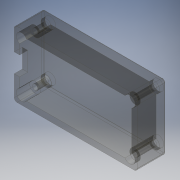
# Autodesk Inventor part: sevo onder
Saved by Autodesk Inventor 2019 (Build 230136000, 136)
## iProperties
Created: 2021-01-16
Part Number: sevo onder
Material: Glass
Document SubType Name: Modeling
Designer: CS
Density: 2.18 g/cm^3
Appearance: Clear servo black(1)
Author: CS
Autodesk Inventor part; units mm, degrees
ref_plane "YZ Plane" through (0, 0, 0) normal (1, 0, 0) x (0, 1, 0)
ref_plane "XZ Plane" through (0, 0, 0) normal (0, 1, 0) x (-1, 0, 0)
ref_plane "XY Plane" through (0, 0, 0) normal (0, 0, 1) x (1, 0, 0)
sketch "Sketch1" plane through (0, 0, 0) normal (0, 0, 1) x (1, 0, 0)
  line L0 (11.375, -6.1) -> (-11.375, -6.1)
  line L1 (-11.375, -6.1) -> (-11.375, 6.1)
  line L2 (-11.375, 6.1) -> (11.375, 6.1)
  line L3 (11.375, 6.1) -> (11.375, -6.1)
  line L4 (11.375, -6.1) -> (-11.375, 6.1) construction
  line L5 (-11.375, -6.1) -> (11.375, 6.1) construction
  point P0 (0, 0)
  dimension "d0" = 12.2
  dimension "d1" = 22.75
  constraints: 12 end point, 2 midpoint, 2 parallel, 1 horizontal, 1 perpendicular
  measures "d0" distance of L2.end L0.start
  measures "d1" distance of L1.end L2.end
extrude "Extrusion1" add sketch "Sketch1" along normal blind 5.3
fillet "Fillet1" radius 0.5 4 edges at (-11.375, 6.1, 2.65) (-11.375, -6.1, 2.65) (11.375, -6.1, 2.65) (11.375, 6.1, 2.65)
fillet "Fillet1" radius 0.25 4 edges at (0, -6.1, 0) (-11.375, 0, 0) (0, 6.1, 0) (11.375, 0, 0)
sketch "Sketch2" plane through (0, 0, 5.3) normal (0, 0, 1) x (1, 0, 0)
  line L0 (10.375, -5) -> (-10.375, -5)
  line L1 (-10.375, -5) -> (-10.375, 5)
  line L2 (-10.375, 5) -> (10.375, 5)
  line L3 (10.375, 5) -> (10.375, -5)
  line L4 (10.375, -5) -> (-10.375, 5) construction
  line L5 (-10.375, -5) -> (10.375, 5) construction
  line L6 (10.875, 6.1) -> (-10.875, 6.1) projected
  line L7 (-11.375, 5.6) -> (-11.375, -5.6) projected
  line L8 (-11.375, -5.6) -> (-11.375, 5.6) projected
  line L9 (-10.375, -1.75) -> (-11.375, -1.75)
  line L10 (-11.375, -1.75) -> (-11.375, 1.75)
  line L11 (-11.375, 1.75) -> (-10.375, 1.75)
  line L12 (-10.375, 1.75) -> (-10.375, -1.75)
  line L13 (10, -4.5) -> (-10, -4.5) construction
  line L14 (-10, -4.5) -> (-10, 4.5) construction
  line L15 (-10, 4.5) -> (10, 4.5) construction
  line L16 (10, 4.5) -> (10, -4.5) construction
  line L17 (10, -4.5) -> (-10, 4.5) construction
  line L18 (-10, -4.5) -> (10, 4.5) construction
  circle A0 centre (-10, 4.5) radius 0.5
  circle A1 centre (10, 4.5) radius 0.5
  circle A2 centre (-10, -4.5) radius 0.5
  circle A3 centre (10, -4.5) radius 0.5
  circle A4 centre (-10, 4.5) radius 1
  circle A5 centre (10, 4.5) radius 1
  circle A6 centre (-10, -4.5) radius 1
  circle A7 centre (10, -4.5) radius 1
  point P0 (0, 0)
  point P1 (-11.375, 0)
  point P2 (0, 0)
  point P3 (-11.375, 0)
  point P4 (0, 0)
  dimension "d6" = 1.1
  dimension "d7" = 1
  dimension "d8" = 3.5
  dimension "d9" = 20
  dimension "d10" = 9
  dimension "d11" = 1
  dimension "d12" = 2
  constraints: 32 end point, 8 centre point, 8 coincident, 8 midpoint, 6 equal radius, 6 parallel, 3 horizontal, 3 perpendicular, 2 horizontal alignment, 2 point on line
  measures "d6" distance between parallel lines of L6 L2
  measures "d7" distance between parallel lines of L7 L1
  measures "d8" distance between parallel lines of L9 L11
  measures "d9" distance of L14.end L15.end
  measures "d10" distance of L15.end L13.start
  measures "d11" diameter of A0
  measures "d12" diameter of A4
extrude "Extrusion2" cut sketch "Sketch2" against normal blind 4.5 contours L0 A3 L3 | L0 A7 L3 A3 | A3 L3 | L0 A6 L1 A4 L2 A5 L3 A7 | L0 A2 L1 A6 | L0 L1 A2 | A2 L1 | A5 L2 A1 L3 | A1 L3 | A1 L2 L3 | A4 L1 A0 L2 | A0 L1 L2 | A0 L1 picked at (10.2274, -3.7042) picked at (10.11, -4.5904) picked at (-9.1814, -4.3794) picked at (-10.0833, -4.5) picked at (10.2274, 3.7042) picked at (10.1829, 4.6853) picked at (-9.1814, 4.3794) picked at (-10.0875, 4.5371)
extrude "Extrusion3" cut sketch "Sketch2" against normal through all contours A3 L3 | L3 A3 | A2 L1 | A2 L1 | A1 L3 | L3 A1 | A0 L1 | A0 L1
extrude "Extrusion4" add sketch "Sketch2" along normal blind 2 from surface at -4.5 contours A6 L1 A2 L0 | L0 A2 L1 A6 | L0 L1 A2 | A4 L1 A0 L2 | L2 L1 A0 A4 | A0 L1 L2
extrude "Extrusion5" cut sketch "Sketch2" against normal up to surface (2.5 mm away) contours A6 L1 A2 L0 | L0 A2 L1 A6 | L0 L1 A2 | A4 L1 A0 L2 | L2 L1 A0 A4 | A0 L1 L2
extrude "Extrusion6" add sketch "Sketch2" along normal blind 3.5 from surface at -4.5 contours L3 A3 A7 L0 | L0 A3 L3 | L0 A7 L3 A3 | A5 L2 A1 L3 | L3 A1 L2 A5 | A1 L2 L3
extrude "Extrusion7" cut sketch "Sketch2" against normal up to surface (1 mm away) contours L3 A3 A7 L0 | L0 A3 L3 | L0 A7 L3 A3 | A5 L2 A1 L3 | L3 A1 L2 A5 | A1 L2 L3
extrude "Extrusion8" cut sketch "Sketch2" against normal blind 1.5 contours L9 L7 L11 L1
extrude "Extrusion9" cut sketch "Sketch2" along normal blind 0.75 from surface at -5.3 contours L3 A3 A7 L0 | L0 A3 L3 | L0 A7 L3 A3 | A6 L1 A2 L0 | L0 A2 L1 A6 | L0 L1 A2 | A5 L2 A1 L3 | L3 A1 L2 A5 | A1 L2 L3 | A4 L1 A0 L2 | L2 L1 A0 A4 | A0 L1 L2
body "Solid1"
